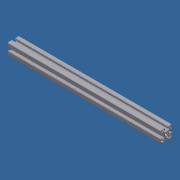
# Autodesk Inventor part: lower side rail
Saved by Autodesk Inventor 2012 (Build 160160000, 160)
## iProperties
Created: 2012-03-15
Part Number: lower side rail
Material: Aluminum-6061
Document SubType Name: Modeling
Designer: Ed
Density: 2.71 g/cm^3
Mass: 785.461 g
Surface Area: 2730.12 cm^2
Volume: 289.838 cm^3
Translation Standard: STEP AP203
FileName: 3842529339_032914984.stp
PreProcessor: ACIS
PostProcessor: Build: 160, Release: 2012 RTM - Date: Tue 03/01/2011
Sent Units: millimeter
Uncertainty: 1e-06
Author: Ed
Autodesk Inventor part; units mm, degrees
ref_plane "YZ Plane" through (0, 0, 0) normal (1, 0, 0) x (0, 1, 0)
ref_plane "XZ Plane" through (0, 0, 0) normal (0, 1, 0) x (-1, 0, 0)
ref_plane "XY Plane" through (0, 0, 0) normal (0, 0, 1) x (1, 0, 0)
sketch "Sketch1" plane through (0, 0, 0) normal (1, 0, 0) x (0, 1, 0)
  line L0 (0, 12.1716) -> (0, 0)
  line L1 (0, 0) -> (-3.9642, -3.9642)
  line L2 (-3.9642, -3.9642) -> (-6.5, -3.9642)
  line L3 (-6.5, -3.9642) -> (-6.5, 1.0858)
  line L4 (-6.5, 1.0858) -> (-11, 1.0858)
  line L5 (-11, 1.0858) -> (-11, 0.2858)
  line L6 (-11, 0.2858) -> (-12.5, 0.2858)
  line L7 (-12.5, 0.2858) -> (-12.5, -10.9142)
  arc A0 (-12.5, -10.9142) -> (-9.5, -13.9142) centre (-9.5, -10.9142) ccw
  line L8 (-9.5, -13.9142) -> (1.7, -13.9142)
  line L9 (1.7, -13.9142) -> (1.7, -12.4142)
  line L10 (1.7, -12.4142) -> (2.5, -12.4142)
  line L11 (2.5, -12.4142) -> (2.5, -7.9142)
  line L12 (2.5, -7.9142) -> (-2.55, -7.9142)
  line L13 (-2.55, -7.9142) -> (-2.55, -5.3784)
  line L14 (-2.55, -5.3784) -> (1.4142, -1.4142)
  line L15 (1.4142, -1.4142) -> (13.5858, -1.4142)
  line L16 (13.5858, -1.4142) -> (17.55, -5.3784)
  line L17 (17.55, -5.3784) -> (17.55, -7.9142)
  line L18 (17.55, -7.9142) -> (12.5, -7.9142)
  line L19 (12.5, -7.9142) -> (12.5, -12.4142)
  line L20 (12.5, -12.4142) -> (13.3, -12.4142)
  line L21 (13.3, -12.4142) -> (13.3, -13.9142)
  line L22 (13.3, -13.9142) -> (24.5, -13.9142)
  arc A1 (24.5, -13.9142) -> (27.5, -10.9142) centre (24.5, -10.9142) ccw
  line L23 (27.5, -10.9142) -> (27.5, 0.2858)
  line L24 (27.5, 0.2858) -> (26, 0.2858)
  line L25 (26, 0.2858) -> (26, 1.0858)
  line L26 (26, 1.0858) -> (21.5, 1.0858)
  line L27 (21.5, 1.0858) -> (21.5, -3.9642)
  line L28 (21.5, -3.9642) -> (18.9642, -3.9642)
  line L29 (18.9642, -3.9642) -> (15, 0)
  line L30 (15, 0) -> (15, 12.1716)
  line L31 (15, 12.1716) -> (18.9642, 16.1358)
  line L32 (18.9642, 16.1358) -> (21.5, 16.1358)
  line L33 (21.5, 16.1358) -> (21.5, 11.0858)
  line L34 (21.5, 11.0858) -> (26, 11.0858)
  line L35 (26, 11.0858) -> (26, 11.8858)
  line L36 (26, 11.8858) -> (27.5, 11.8858)
  line L37 (27.5, 11.8858) -> (27.5, 23.0858)
  arc A2 (27.5, 23.0858) -> (24.5, 26.0858) centre (24.5, 23.0858) ccw
  line L38 (24.5, 26.0858) -> (13.3, 26.0858)
  line L39 (13.3, 26.0858) -> (13.3, 24.5858)
  line L40 (13.3, 24.5858) -> (12.5, 24.5858)
  line L41 (12.5, 24.5858) -> (12.5, 20.0858)
  line L42 (12.5, 20.0858) -> (17.55, 20.0858)
  line L43 (17.55, 20.0858) -> (17.55, 17.55)
  line L44 (17.55, 17.55) -> (13.5858, 13.5858)
  line L45 (13.5858, 13.5858) -> (1.4142, 13.5858)
  line L46 (1.4142, 13.5858) -> (-2.55, 17.55)
  line L47 (-2.55, 17.55) -> (-2.55, 20.0858)
  line L48 (-2.55, 20.0858) -> (2.5, 20.0858)
  line L49 (2.5, 20.0858) -> (2.5, 24.5858)
  line L50 (2.5, 24.5858) -> (1.7, 24.5858)
  line L51 (1.7, 24.5858) -> (1.7, 26.0858)
  line L52 (1.7, 26.0858) -> (-9.5, 26.0858)
  arc A3 (-9.5, 26.0858) -> (-12.5, 23.0858) centre (-9.5, 23.0858) ccw
  line L53 (-12.5, 23.0858) -> (-12.5, 11.8858)
  line L54 (-12.5, 11.8858) -> (-11, 11.8858)
  line L55 (-11, 11.8858) -> (-11, 11.0858)
  line L56 (-11, 11.0858) -> (-6.5, 11.0858)
  line L57 (-6.5, 11.0858) -> (-6.5, 16.1358)
  line L58 (-6.5, 16.1358) -> (-3.9642, 16.1358)
  line L59 (-3.9642, 16.1358) -> (0, 12.1716)
  line L60 (-0.5, 24.5858) -> (-0.5, 21.5858)
  line L61 (-0.5, 21.5858) -> (-4.25, 21.5858)
  line L62 (-4.25, 21.5858) -> (-4.25, 20.5858)
  arc A4 (-7, 17.8358) -> (-4.25, 20.5858) centre (-7, 20.5858) ccw
  line L63 (-7, 17.8358) -> (-8, 17.8358)
  line L64 (-8, 17.8358) -> (-8, 14.0858)
  line L65 (-8, 14.0858) -> (-11, 14.0858)
  line L66 (-11, 14.0858) -> (-11, 20.5858)
  line L67 (-11, 20.5858) -> (-9.75, 20.5858)
  arc A5 (-7, 23.3358) -> (-9.75, 20.5858) centre (-7, 20.5858) ccw
  line L68 (-7, 23.3358) -> (-7, 24.5858)
  line L69 (-7, 24.5858) -> (-0.5, 24.5858)
  line L70 (26, 14.0858) -> (23, 14.0858)
  line L71 (23, 14.0858) -> (23, 17.8358)
  line L72 (23, 17.8358) -> (22, 17.8358)
  arc A6 (19.25, 20.5858) -> (22, 17.8358) centre (22, 20.5858) ccw
  line L73 (19.25, 20.5858) -> (19.25, 21.5858)
  line L74 (19.25, 21.5858) -> (15.5, 21.5858)
  line L75 (15.5, 21.5858) -> (15.5, 24.5858)
  line L76 (15.5, 24.5858) -> (22, 24.5858)
  line L77 (22, 24.5858) -> (22, 23.3358)
  arc A7 (24.75, 20.5858) -> (22, 23.3358) centre (22, 20.5858) ccw
  line L78 (24.75, 20.5858) -> (26, 20.5858)
  line L79 (26, 20.5858) -> (26, 14.0858)
  line L80 (15.5, -12.4142) -> (15.5, -9.4142)
  line L81 (15.5, -9.4142) -> (19.25, -9.4142)
  line L82 (19.25, -9.4142) -> (19.25, -8.4142)
  arc A8 (22, -5.6642) -> (19.25, -8.4142) centre (22, -8.4142) ccw
  line L83 (22, -5.6642) -> (23, -5.6642)
  line L84 (23, -5.6642) -> (23, -1.9142)
  line L85 (23, -1.9142) -> (26, -1.9142)
  line L86 (26, -1.9142) -> (26, -8.4142)
  line L87 (26, -8.4142) -> (24.75, -8.4142)
  arc A9 (22, -11.1642) -> (24.75, -8.4142) centre (22, -8.4142) ccw
  line L88 (22, -11.1642) -> (22, -12.4142)
  line L89 (22, -12.4142) -> (15.5, -12.4142)
  line L90 (9.761, 0.8858) -> (9.4937, 1.5005)
  arc A10 (5.5063, 1.5005) -> (9.4937, 1.5005) centre (7.5, 6.0858) ccw
  line L91 (5.5063, 1.5005) -> (5.239, 0.8858)
  line L92 (5.239, 0.8858) -> (2.3, 0.8858)
  line L93 (2.3, 0.8858) -> (2.3, 3.8248)
  line L94 (2.3, 3.8248) -> (2.9147, 4.092)
  arc A11 (2.9147, 8.0795) -> (2.9147, 4.092) centre (7.5, 6.0858) ccw
  line L95 (2.9147, 8.0795) -> (2.3, 8.3468)
  line L96 (2.3, 8.3468) -> (2.3, 11.2858)
  line L97 (2.3, 11.2858) -> (5.239, 11.2858)
  line L98 (5.239, 11.2858) -> (5.5063, 10.6711)
  arc A12 (9.4937, 10.6711) -> (5.5063, 10.6711) centre (7.5, 6.0858) ccw
  line L99 (9.4937, 10.6711) -> (9.761, 11.2858)
  line L100 (9.761, 11.2858) -> (12.7, 11.2858)
  line L101 (12.7, 11.2858) -> (12.7, 8.3468)
  line L102 (12.7, 8.3468) -> (12.0853, 8.0795)
  arc A13 (12.0853, 4.092) -> (12.0853, 8.0795) centre (7.5, 6.0858) ccw
  line L103 (12.0853, 4.092) -> (12.7, 3.8248)
  line L104 (12.7, 3.8248) -> (12.7, 0.8858)
  line L105 (12.7, 0.8858) -> (9.761, 0.8858)
  line L106 (-11, -1.9142) -> (-8, -1.9142)
  line L107 (-8, -1.9142) -> (-8, -5.6642)
  line L108 (-8, -5.6642) -> (-7, -5.6642)
  arc A14 (-4.25, -8.4142) -> (-7, -5.6642) centre (-7, -8.4142) ccw
  line L109 (-4.25, -8.4142) -> (-4.25, -9.4142)
  line L110 (-4.25, -9.4142) -> (-0.5, -9.4142)
  line L111 (-0.5, -9.4142) -> (-0.5, -12.4142)
  line L112 (-0.5, -12.4142) -> (-7, -12.4142)
  line L113 (-7, -12.4142) -> (-7, -11.1642)
  arc A15 (-9.75, -8.4142) -> (-7, -11.1642) centre (-7, -8.4142) ccw
  line L114 (-9.75, -8.4142) -> (-11, -8.4142)
  line L115 (-11, -8.4142) -> (-11, -1.9142)
  constraints: 232 end point, 50 horizontal, 50 vertical, 32 point on circle, 16 centre point, 180 other
extrude "Extrusion1" add sketch "Sketch1" along normal blind 521.975
body "Solid2"
